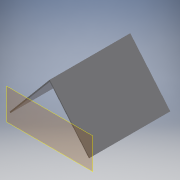
# Autodesk Inventor part: Haus_Dach
Saved by Autodesk Inventor 2017 (Build 210142000, 142)
## iProperties
Created: 2017-06-01
Part Number: Haus_Dach
Material: Generic
Document SubType Name: Modeling
Designer: Fake
Density: 1 g/cm^3
Appearance: Default
Author: Fake
Autodesk Inventor part; units mm, degrees
ref_plane "YZ Plane" through (0, 0, 0) normal (1, 0, 0) x (0, 1, 0)
ref_plane "XZ Plane" through (0, 0, 0) normal (0, 1, 0) x (-1, 0, 0)
ref_plane "Arbeitsebene1" through (-1284.1409, -3575, 3900) normal (0, -1, 0) x (1, 0, 0)
sketch "Skizze1" plane through (-1284.1409, -3575, 3900) normal (0, -1, 0) x (1, 0, 0)
  line L0 (1990.078, 2180) -> (3070.078, 2180) projected
  line L1 (3070.078, 2180) -> (3070.078, 1000) projected
  line L2 (3070.078, 1000) -> (1990.078, 1000) projected
  line L3 (1990.078, 1000) -> (1990.078, 2180) projected
  line L4 (5324.6225, 2180) -> (5324.6225, 1000) projected
  line L5 (5324.6225, 1000) -> (4244.6225, 1000) projected
  line L6 (4244.6225, 1000) -> (4244.6225, 2180) projected
  line L7 (4244.6225, 2180) -> (5324.6225, 2180) projected
  line L8 (1486.4055, 2500) -> (0, 728.5709) projected
  line L9 (0, 0) -> (0, 728.5709) projected
  line L10 (0, 0) -> (6964.1409, 0) projected
  line L11 (6964.1409, 0) -> (6964.1409, 728.5709) projected
  line L12 (6964.1409, 728.5709) -> (5477.7354, 2500) projected
  line L13 (1486.4055, 2500) -> (5477.7354, 2500) projected
  line L14 (0, 728.5709) -> (3482.0704, 4878.3408)
  line L15 (6964.1409, 728.5709) -> (3482.0704, 4878.3408)
  line L16 (-76.6044, 792.8496) -> (3482.0704, 5033.9132)
  line L17 (3482.0704, 5033.9132) -> (7029.4112, 806.3571)
  line L18 (0, 728.5709) -> (-76.6044, 792.8496)
  line L19 (6964.1409, 728.5709) -> (7029.4112, 806.3571)
  dimension "d0" = 100
  constraints: 12 end point, 2 perpendicular, 2 point on line, 1 other
  measures "d0" distance between parallel lines of L14 L16
ref_plane "Arbeitsebene2" through (-1284.1409, 3575, 3900) normal (0, 1, 0) x (0, 0, 1)
extrude "Extrusion1" add sketch "Skizze1" against normal up to surface (7150 mm away) contours L8 L18 L16 L17 L19 L12 L15 L14
